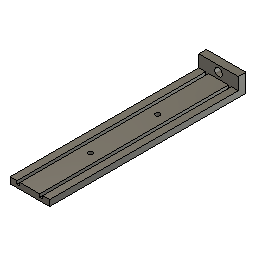
System E (Autodesk Fusion 360 archive; units mm, degrees)
design "İmkansızlar Yan Taraf Kapatıcı"
Autodesk Fusion 360 part; units mm, degrees
sketch "Eskiz1" plane through (0, 0, 0) normal (0, 1, 0) x (1, 0, 0)
  line L0 (0, 0) -> (26, 0)
  line L1 (26, 0) -> (26, -124)
  line L2 (26, -124) -> (0, -124)
  line L3 (0, -124) -> (0, 0)
  line L4 (4.5, 0) -> (6.5, 0)
  line L5 (6.5, 0) -> (6.5, -124)
  line L6 (6.5, -124) -> (4.5, -124)
  line L7 (4.5, -124) -> (4.5, 0)
  line L8 (19.5, 0) -> (21.5, 0)
  line L9 (21.5, 0) -> (21.5, -124)
  line L10 (21.5, -124) -> (19.5, -124)
  line L11 (19.5, -124) -> (19.5, 0)
  line L12 (0, 0) -> (26, 0)
  line L13 (26, 0) -> (26, 5)
  line L14 (26, 5) -> (0, 5)
  line L15 (0, 5) -> (0, 0)
  line L16 (0, -124) -> (26, -124)
  line L17 (26, -124) -> (26, -129)
  line L18 (26, -129) -> (0, -129)
  line L19 (0, -129) -> (0, -124)
  dimension "d1" = 26
  dimension "d2" = 124
  dimension "d3" = 2
  dimension "d4" = 4.5
  dimension "d5" = 2
  dimension "d6" = 13
  dimension "d11" = 5
  dimension "d18" = 5
  constraint horizontal L0
  constraint vertical L1
  constraint horizontal L2
  constraint vertical L3
  constraint coincident L0.start L3.end
  constraint horizontal L4
  constraint vertical L5
  constraint horizontal L6
  constraint vertical L7
  constraint coincident L0 L4.start
  constraint horizontal L8
  constraint vertical L9
  constraint horizontal L10
  constraint vertical L11
  constraint coincident L0 L8.start
  constraint horizontal L12
  constraint vertical L13
  constraint horizontal L14
  constraint vertical L15
  constraint horizontal L16
  constraint vertical L17
  constraint horizontal L18
  constraint vertical L19
  measures "d1" distance of L0.start L0.end
  measures "d2" distance of L0.start L2.end
  measures "d3" distance of L4.start L4.end
  measures "d4" distance of L0.start L4.start
  measures "d5" distance of L8.start L8.end
  measures "d6" distance of L4.end L8.start
  measures "d11" distance of L0.start L14.end
  measures "d18" distance of L2.end L18.end
extrude "Ekstrüde Et1" add sketch "Eskiz1" along normal blind 2 contours L0 L2 L4 L5 L6 L7 L12 L16 | L0 L2 L8 L9 L10 L11 L12 L16 makes body 1 at (6.5, 0.6667, 41.3333) makes body 2 at (21.5, 0.6667, 41.3333)
extrude "Ekstrüde Et2" add sketch "Eskiz1" along normal blind 4 contours L0 L2 L3 L7 L12 L16 | L0 L2 L5 L11 L12 L16 | L0 L1 L2 L9 L12 L16 bodies 1 2
extrude "Ekstrüde Et3" add sketch "Eskiz1" along normal blind 12 contours L0 L4 L8 L12 L13 L14 L15 bodies 1
sketch "Eskiz2" plane through (0, 0, -5) normal (0, 0, -1) x (-1, 0, 0)
  line L0 (-26, 0) -> (0, 0)
  line L1 (0, 0) -> (0, 12)
  line L2 (0, 12) -> (-26, 12)
  line L3 (-26, 12) -> (-26, 0)
  circle A0 centre (-13, 8) radius 2.5
  dimension "d14" = 5
  dimension "d15" = 4
  measures "d14" diameter of A0
  measures "d15" distance of L2 A0.centre
extrude "Ekstrüde Et4" cut sketch "Eskiz2" against normal blind 6 contours A0 bodies 1
sketch "Eskiz3" plane through (0, 4, 0) normal (0, 1, 0) x (-1, 0, 0)
  line L0 (-6.5, 0) -> (-6.5, 124)
  line L1 (-6.5, 124) -> (-19.5, 124)
  line L2 (-19.5, 124) -> (-19.5, 0)
  line L3 (-19.5, 0) -> (-6.5, 0)
  circle A0 centre (-13, 84) radius 1.5
  circle A1 centre (-13, 40) radius 1.5
  dimension "d19" = 3
  dimension "d20" = 3
  dimension "d21" = 40
  dimension "d22" = 40
  measures "d19" diameter of A0
  measures "d20" diameter of A1
  measures "d21" distance of L3 A1.centre
  measures "d22" distance of L1 A0.centre
extrude "Ekstrüde Et5" cut sketch "Eskiz3" against normal blind 15 contours A0 | A1 bodies 1

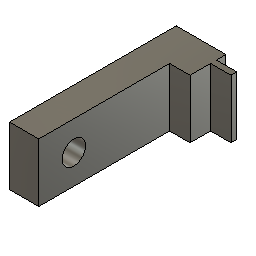
design "İmkansızlar Birleştirme Parçası"
Autodesk Fusion 360 part; units mm, degrees
sketch "Eskiz1" plane through (0, 0, 0) normal (0, 1, 0) x (1, 0, 0)
  line L0 (0, -11.5) -> (0, 0)
  line L1 (0, 0) -> (15, 0)
  line L2 (15, 0) -> (15, -45)
  line L3 (15, -45) -> (0, -45)
  line L4 (0, -45) -> (0, 0)
  dimension "d3" = 15
  dimension "d4" = 45
  constraint vertical L0
  constraint coincident L0.end L1.start
  constraint horizontal L1
  constraint vertical L2
  constraint horizontal L3
  constraint vertical L4
  measures "d3" distance of L0.end L1.end
  measures "d4" distance of L0.end L3.end
extrude "Ekstrüde Et1" add sketch "Eskiz1" along normal blind 20
sketch "Eskiz2" plane through (0, 0, 0) normal (-1, 0, 0) x (0, 0, 1)
  line L0 (0, 0) -> (45, 0)
  line L1 (45, 0) -> (45, 20)
  line L2 (45, 20) -> (0, 20)
  line L3 (0, 20) -> (0, 0)
  line L4 (0, 0) -> (15, 0)
  line L5 (15, 0) -> (15, 20)
  line L6 (15, 20) -> (0, 20)
  line L7 (0, 20) -> (0, 0)
  circle A0 centre (33, 10) radius 4
  point P0 (37, 10)
  dimension "d7" = 15
  dimension "d8" = 20
  dimension "d9" = 8
  dimension "d10" = 8
  constraint horizontal L4
  constraint vertical L5
  constraint horizontal L6
  constraint vertical L7
  constraint coincident L0.start L3.end
  constraint coincident A0 P0
  measures "d7" distance of L0.start L4.end
  measures "d8" distance of L0.start L2.end
  measures "d9" diameter of A0
  measures "d10" distance of L1 P0
extrude "Ekstrüde Et2" cut sketch "Eskiz2" against normal blind 20 contours A0
sketch "Eskiz4" plane through (15, 0, 0) normal (1, 0, 0) x (0, 0, -1)
  circle A0 centre (-33, 10) radius 4
  line L0 (-45, 0) -> (0, 0)
  line L1 (0, 0) -> (0, 20)
  line L2 (0, 20) -> (-45, 20)
  line L3 (-45, 20) -> (-45, 0)
  line L4 (0, 0) -> (-10, 0)
  line L5 (-10, 0) -> (-10, 20)
  line L6 (-10, 20) -> (0, 20)
  line L7 (0, 20) -> (0, 0)
  dimension "d22" = 10
  constraint horizontal L4
  constraint vertical L5
  constraint horizontal L6
  constraint vertical L7
  constraint coincident L0.end L1.start
  measures "d22" distance of L0.end L4.end
extrude "Ekstrüde Et6" add sketch "Eskiz4" along normal blind 7 contours L0 L1 L2 L4 L5 L6 L7
sketch "Eskiz5" plane through (0, 0, 0) normal (0, 0, -1) x (-1, 0, 0)
  line L0 (-22, 0) -> (0, 0)
  line L1 (0, 0) -> (0, 20)
  line L2 (0, 20) -> (-22, 20)
  line L3 (-22, 20) -> (-22, 0)
  line L4 (-22, 0) -> (-15, 0)
  line L5 (-15, 0) -> (-15, 20)
  line L6 (-15, 20) -> (-22, 20)
  line L7 (-22, 20) -> (-22, 0)
  dimension "d25" = 7
  dimension "d26" = 20
  constraint horizontal L4
  constraint vertical L5
  constraint horizontal L6
  constraint vertical L7
  constraint coincident L0.start L3.end
  measures "d25" distance of L0.start L4.end
  measures "d26" distance of L0.start L2.end
extrude "Ekstrüde Et7" add sketch "Eskiz5" along normal blind 12 contours L0 L2 L3 L4 L5 L6 L7
extrude "Ekstrüde Et9" cut 1 faces at (0, 10, 9.6667) along direction (1, 0, 0) blind 5
sketch "Eskiz7" plane through (22, 0, 0) normal (1, 0, 0) x (0, 0, -1)
  line L0 (12, 20) -> (-10, 20)
  line L1 (-10, 20) -> (-10, 0)
  line L2 (-10, 0) -> (12, 0)
  line L3 (12, 0) -> (12, 20)
  line L4 (6.7308, 20) -> (8.7308, 20)
  line L5 (8.7308, 20) -> (8.7308, 0)
  line L6 (8.7308, 0) -> (6.7308, 0)
  line L7 (6.7308, 0) -> (6.7308, 20)
  dimension "d36" = 2
  constraint horizontal L4
  constraint vertical L5
  constraint horizontal L6
  constraint vertical L7
  constraint coincident L0 L4.start
  measures "d36" distance of L4.start L4.end
extrude "Ekstrüde Et10" add sketch "Eskiz7" along normal blind 7 contours L0 L2 L4 L5 L6 L7
extrude "Ekstrüde Et11" add 1 faces at (11.6667, 13.3333, 0) along direction (0, 0, -1) blind 12
extrude "Ekstrüde Et12" cut 1 faces at (17.3333, 6.6667, 10) along direction (0, 0, -1) blind 9.731

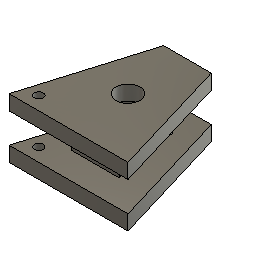
design "Bobin Birleşik"
Autodesk Fusion 360 part; units mm, degrees
sketch "Eskiz1" plane through (0, 0, 0) normal (0, 1, 0) x (1, 0, 0)
  line L0 (0, 0) -> (40, 0)
  line L1 (40, 0) -> (40, -40)
  line L2 (40, -40) -> (0, -40)
  line L3 (0, -40) -> (0, 0)
  line L4 (12, 0) -> (35, 0)
  line L5 (35, -40) -> (12, -40)
  line L6 (12, -40) -> (12, 0)
  line L7 (28, 0) -> (28, -40)
  line L8 (12, 0) -> (0, -40)
  line L9 (28, 0) -> (40, -40)
  circle A0 centre (20, -20) radius 4
  point P0 (12, 0)
  point P1 (28, 0)
  dimension "d1" = 40
  dimension "d2" = 40
  dimension "d3" = 12
  dimension "d4" = 12
  dimension "d5" = 40
  dimension "d23" = 8
  constraint horizontal L0
  constraint vertical L1
  constraint horizontal L2
  constraint vertical L3
  constraint coincident L0.start L3.end
  constraint coincident L0 P0
  constraint coincident L0 P1
  constraint horizontal L4
  constraint horizontal L5
  constraint vertical L6
  constraint coincident L2 L5.start
  constraint coincident P0 L4.start
  constraint vertical L7
  constraint coincident P1 L7.start
  measures "d1" distance of L0.start L0.end
  measures "d2" distance of L0.start L2.end
  measures "d3" distance of L0.start L4.start
  measures "d4" distance of L0.end P1
  measures "d5" distance of P1 L7.end
  measures "d23" diameter of A0
extrude "Ekstrüde Et1" add sketch "Eskiz1" along normal blind 5 contours L0 L2 L4 L5 L6 L7 | L2 L6 L8 | L2 L5 L7 L9 | A0 makes body 1
sketch "Eskiz2" plane through (0, 5, 0) normal (0, 1, 0) x (-1, 0, 0)
  line L0 (-12, 0) -> (0, 40)
  line L1 (0, 40) -> (-40, 40)
  line L2 (-40, 40) -> (-28, 0)
  line L3 (-28, 0) -> (-12, 0)
  line L4 (-12, 0) -> (-28, 0)
  line L5 (-28, 0) -> (-28, 40)
  line L6 (-28, 40) -> (-12, 40)
  line L7 (-12, 40) -> (-12, 0)
  line L8 (-12, 31) -> (-28, 31)
  line L9 (-16, 9) -> (-12, 31)
  line L10 (-24, 9) -> (-28, 31)
  line L11 (-16, 9) -> (-24, 9)
  circle A0 centre (-5.5, 35.5) radius 1.5
  point P0 (-16, 9)
  point P1 (-24, 9)
  point P2 (-12, 35.5)
  point P3 (-5.5, 35.5)
  dimension "d8" = 16
  dimension "d9" = 40
  dimension "d16" = 4
  dimension "d17" = 4
  dimension "d18" = 9
  dimension "d19" = 9
  dimension "d20" = 9
  dimension "d33" = 6.5
  dimension "d34" = 4.5
  dimension "d35" = 3
  constraint horizontal L4
  constraint vertical L5
  constraint horizontal L6
  constraint vertical L7
  constraint coincident L0.start L3.end
  constraint coincident L7 L8.start
  constraint coincident L5 L8.end
  constraint perpendicular L5 L8
  constraint coincident P0 L9.start
  constraint coincident P1 L10.start
  constraint coincident L7 P2
  constraint coincident P3 A0.centre
  measures "d8" distance of L0.start L2.end
  measures "d9" distance of L0.start L6.end
  measures "d16" distance of L7 P0
  measures "d17" distance of L5 P1
  measures "d18" distance of L4 P1
  measures "d19" distance of L4 P0
  measures "d20" distance of L6 L8
  measures "d33" distance of P2 P3
  measures "d34" distance of L8 P2
  measures "d35" diameter of A0
copy_body "CopyPasteBodies1" bodies 1 makes body 2
extrude "Ekstrüde Et4" add sketch "Eskiz2" along normal blind 10 contours L8 L9 L10 L11 bodies 1
move_body "Taşı1" bodies 2 to x (1, 0, 0) y (0, 1, 0) z (0, 0, 1) at (0, 15, 0)
extrude "Ekstrüde Et5" cut sketch "Eskiz1" along normal blind 25 contours A0 bodies 1 2
extrude "Ekstrüde Et6" cut sketch "Eskiz2" along normal blind 19 and the other way blind 8.5 contours A0 bodies 1 2
